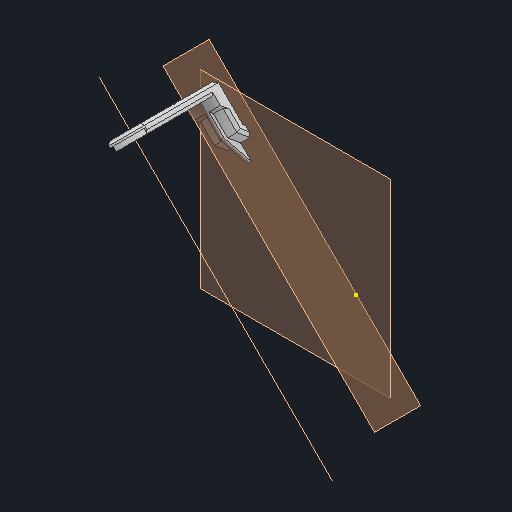
# Autodesk Inventor part: Venstre arm
Saved by Autodesk Inventor 2026.1 (Build 301233020, 233B)
## iProperties
Created: 2025-09-26
Part Number: Venstre arm
Material: Generic
Document SubType Name: Modeling
Designer: Malthe Sennels
Density: 1 g/cm^3
Appearance: Default
Author: Malthe Sennels
Autodesk Inventor part; units mm, degrees
ref_plane "YZ Plane" through (0, 0, 0) normal (1, 0, 0) x (0, 1, 0)
ref_plane "XZ Plane" through (0, 0, 0) normal (0, 1, 0) x (-1, 0, 0)
ref_plane "XY Plane" through (0, 0, 0) normal (0, 0, 1) x (1, 0, 0)
ref_plane "Work Plane1" through (0, 0, 0) normal (0, 0, 1) x (1, 0, 0)
sketch "Sketch1" plane through (0, 0, 0) normal (0, 0, 1) x (1, 0, 0)
  line L0 (-18.9164, 56.7911) -> (-19.9626, 56.4354) projected
  arc A0 (-12.4369, -46.9155) -> (-18.9164, 56.7911) centre (-94.7078, 0) ccw projected
  line L1 (-12.4369, -46.9155) -> (-25.0393, -34.3131) projected
  arc A1 (-25.0393, -34.3131) -> (-32.1104, -34.3131) centre (-28.5748, -37.8487) ccw projected
  line L2 (-32.1104, -34.3131) -> (-60.3946, -62.5974) projected
  arc A2 (-60.3946, -62.5974) -> (-60.3946, -69.6685) centre (-56.8591, -66.1329) ccw projected
  line L3 (-60.3946, -69.6685) -> (-47.7922, -82.2709) projected
  arc A3 (-141.6233, -82.2709) -> (-47.7922, -82.2709) centre (-94.7078, 0) ccw projected
  line L4 (-141.6233, -82.2709) -> (-129.0209, -69.6685) projected
  arc A4 (-129.0209, -69.6685) -> (-129.0209, -62.5974) centre (-132.5564, -66.1329) ccw projected
  line L5 (-129.0209, -62.5974) -> (-157.3052, -34.3131) projected
  arc A5 (-157.3052, -34.3131) -> (-164.3762, -34.3131) centre (-160.8407, -37.8487) ccw projected
  line L6 (-164.3762, -34.3131) -> (-176.9786, -46.9155) projected
  arc A6 (-176.9786, 46.9155) -> (-176.9786, -46.9155) centre (-94.7078, 0) ccw projected
  line L7 (-176.9786, 46.9155) -> (-164.3762, 34.3131) projected
  arc A7 (-164.3762, 34.3131) -> (-157.3052, 34.3131) centre (-160.8407, 37.8487) ccw projected
  line L8 (-157.3052, 34.3131) -> (-129.0209, 62.5974) projected
  arc A8 (-129.0209, 62.5974) -> (-129.0209, 69.6685) centre (-132.5564, 66.1329) ccw projected
  line L9 (-129.0209, 69.6685) -> (-141.6233, 82.2709) projected
  arc A9 (-37.9167, 75.7914) -> (-141.6233, 82.2709) centre (-94.7078, 0) ccw projected
  line L10 (-38.2723, 74.7452) -> (-37.9167, 75.7914) projected
  circle A10 centre (-138.2133, -64.7187) radius 2.25 projected
  circle A11 centre (-159.4265, -43.5055) radius 2.25 projected
  circle A12 centre (-159.4265, 43.5055) radius 2.25 projected
  circle A13 centre (-138.2133, 64.7187) radius 2.25 projected
  circle A14 centre (-51.2022, -64.7187) radius 2.25 projected
  circle A15 centre (-29.989, -43.5055) radius 2.25 projected
  line L11 (-141.6233, 82.2709) -> (-144.5624, 85.21)
  line L12 (-176.9786, 46.9155) -> (-179.9178, 49.8547)
  circle A16 centre (-94.7078, 0) radius 98.723 projected
  arc A17 (-19.9626, 56.4354) -> (-38.2723, 74.7452) centre (-94.7078, 0) ccw projected
  point P0 (0, 0)
  point P1 (-14.9261, 58.1475)
  point P2 (-36.5603, 79.7816)
  point P3 (-193.4308, 0)
  point P4 (-94.7078, -98.723)
  constraints: 4 end point, 2 point on circle, 1 parallel
extrude "Extrusion1" [suppressed]
chamfer "Chamfer1" [suppressed]
ref_plane "Work Plane2" through (-146.6986, 51.9908, -4) normal (0.7071068, 0.7071068, 0) x (0, 0, 1)
sketch "Sketch2" plane through (-146.6986, 51.9908, -4) normal (0.7071068, 0.7071068, 0) x (0, 0, 1)
  line L0 (8, 0) -> (8, -18.8747) projected
  line L1 (8, -18.8747) -> (8, -22.1969) projected
  line L2 (4, 5) -> (8, 5) projected
  line L3 (8, 5) -> (8, 0)
  line L4 (8, 5) -> (19.8525, -22.7909)
  line L5 (19.8525, -22.7909) -> (19.8525, -46.753)
  line L6 (19.8525, -46.753) -> (29.6486, -56.5491)
  line L7 (29.6486, -56.5491) -> (29.6486, -70.8342)
  line L8 (8, -22.1969) -> (9.8525, -24.0494)
  line L9 (8, -22.1969) -> (10.6198, -22.1969) construction
  line L10 (9.8525, -24.0494) -> (9.8525, -51.0381)
  line L11 (9.8525, -51.0381) -> (29.6486, -70.8342)
  line L12 (25.3635, -66.5491) -> (29.6486, -66.5491)
  line L13 (29.6486, -70.8342) -> (9.8525, -70.8342)
  line L14 (9.8525, -70.8342) -> (9.8525, -51.0381)
  line L15 (29.6486, -56.5491) -> (19.8525, -56.5491)
  line L16 (19.8525, -56.5491) -> (19.8525, -46.753)
  line L17 (29.6486, -66.5491) -> (9.8525, -66.5491)
  point P0 (4, 140.4946)
  point P1 (25.3635, -66.5491)
  dimension "d6" = 45
  dimension "d14" = 10
  dimension "d15" = 10
  constraints: 30 end point, 4 perpendicular, 3 point on line, 3 vertical, 2 collinear, 1 equal length, 1 horizontal, 1 parallel
  measures "d6" angle of L8 L9
  measures "d14" distance from line of L6.end L12
  measures "d15" distance between parallel lines of L5 L10
extrude "Extrusion2" add sketch "Sketch2" along normal mid plane 6 contours L3 L4 L5 L16 L15 L7 L12 L11 L10 L8 L1 L0 | L11 L17 L14
sketch "Sketch3" plane through (-144.5772, 54.1121, -4) normal (0.7071068, 0.7071068, 0) x (-0.7071068, 0.7071068, 0)
  line L0 (22.1969, 8) -> (24.0494, 9.8525) projected
  line L1 (24.0494, 9.8525) -> (66.5491, 9.8525) projected
  line L2 (51.0381, 9.8525) -> (66.5491, 25.3635) projected
  line L3 (56.5491, 29.6486) -> (46.753, 19.8525) projected
  line L4 (46.753, 19.8525) -> (43.753, 16.8525)
  line L5 (43.753, 16.8525) -> (21.1499, 16.8525)
  line L6 (21.1499, 16.8525) -> (12.2974, 8)
  line L7 (22.1499, 8) -> (-5, 8) projected
  line L8 (66.5491, 29.6486) -> (56.5491, 29.6486) projected
  line L9 (22.1499, 8) -> (12.2974, 8)
  line L10 (-5, 8) -> (22.1969, 8) projected
  line L11 (66.5491, 9.8525) -> (66.5491, 29.6486) projected
  line L12 (66.5491, 9.8525) -> (24.0494, 9.8525) projected
  line L13 (24.0494, 9.8525) -> (22.1969, 8) projected
  line L14 (22.1969, 8) -> (-5, 8) projected
  line L15 (-5, 8) -> (22.7909, 19.8525) projected
  line L16 (22.7909, 19.8525) -> (56.5491, 19.8525) projected
  line L17 (56.5491, 19.8525) -> (56.5491, 29.6486) projected
  line L18 (56.5491, 29.6486) -> (66.5491, 29.6486) projected
  line L19 (66.5491, 29.6486) -> (66.5491, 9.8525) projected
  point P0 (-140.4946, 4)
  point P1 (70.6913, 29.6486)
  point P2 (66.5491, 25.3635)
  point P3 (56.5491, 29.6486)
  dimension "d10" = 7
  dimension "d11" = 7
  constraints: 8 end point, 2 parallel, 1 collinear, 1 horizontal, 1 point on line, 1 other
  measures "d10" distance between parallel lines of L1 L5
  measures "d11" distance between parallel lines of L6 L0
extrude "Extrusion3" add sketch "Sketch3" along normal blind 18.2 contours L10 L7 L6 L5 L4 L16 L17 L8 L11 L2 L1 L0 | L2 L11 L1
mirror "Mirror1" about plane through (-146.6986, 51.9908, -4) normal (0.7071068, 0.7071068, 0) of "Extrusion3"
sketch "Sketch4" plane through (-171.6942, 106.9677, 25.6486) normal (0, 0, 1) x (0.7071068, 0.7071068, 0)
  point P0 (45.7685, -197.0437)
sketch "Sketch5" plane through (-181.028, 111.7761, 21.3635) normal (-0.7071068, 0.7071068, 0) x (-0.7071068, -0.7071068, 0)
  line L0 (-3.2, -15.511) -> (-3.2, 4.2851) projected
  line L1 (39.2, -15.511) -> (39.2, 4.2851) projected
  line L2 (39.2, 4.2851) -> (-3.2, 4.2851) projected
  line L3 (18, 4.2851) -> (18, 69.2851) construction
  circle A0 centre (18, 69.2851) radius 11
  arc A1 (39.2, 69.2851) -> (-3.2, 69.2851) centre (18, 69.2851) ccw
  line L4 (-3.2, 4.2851) -> (-3.2, 69.2851)
  line L5 (39.2, 4.2851) -> (39.2, 69.2851)
  line L6 (18, 51.2851) -> (4.8, 51.2851)
  line L7 (4.8, 51.2851) -> (-3.2, 59.2851)
  line L8 (18, 51.2851) -> (31.2, 51.2851)
  line L9 (31.2, 51.2851) -> (39.2, 59.2851)
  point P0 (-48.9685, -21.3635)
  point P1 (0, 0)
  point P2 (36, 0)
  dimension "d17" = 22
  dimension "d18" = 65
  dimension "d21" = 135
  dimension "d22" = 18
  dimension "d23" = 8
  constraints: 14 end point, 2 centre point, 2 coincident, 2 midpoint, 2 point on circle, 2 point on line, 2 symmetric about line, 2 vertical, 1 horizontal, 1 parallel, 1 tangent, 2 other
  measures "d17" diameter of A0
  measures "d18" distance of point (18, 4.285) L3.end
  measures "d21" angle of L6 L7
  measures "d22" distance from line of L3.end L6
  measures "d23" distance from line of L4 L6.end
extrude "Extrusion4" add sketch "Sketch5" against normal blind 10
chamfer "Chamfer2" distance 3 angle 45 6 edges at (-186.6848, 91.9771, 111.8486) (-171.6942, 106.9677, 53.2505) (-184.6359, 59.9468, 12.8525) (-154.6545, 89.9281, 12.8525) (-173.5146, 48.8256, 8.4262) (-143.5333, 78.8069, 8.4262)
sketch "Sketch7" plane through (-173.9569, 104.705, 21.3635) normal (0.7071068, -0.7071068, 0) x (0, 0, -1)
  circle A0 centre (-69.2851, -18) radius 11 projected
  line L0 (-69.2851, -18) -> (-10.1777, -18) construction
  line L1 (-51.2851, -18) -> (-51.2851, -30)
  line L2 (-51.2851, -30) -> (-57.2851, -36)
  line L3 (-69.2851, -36) -> (-3.0425, -36) projected
  line L4 (-51.2851, -18) -> (-51.2851, -6)
  line L5 (-51.2851, -6) -> (-57.2851, 0)
  line L6 (-69.2851, -39.2) -> (-69.2851, -36.2) projected
  arc A1 (-69.2851, 0.2) -> (-69.2851, -36.2) centre (-69.2851, -18) ccw projected
  line L7 (-69.2851, 3.2) -> (-69.2851, 0.2) projected
  arc A2 (-69.2851, 3.2) -> (-69.2851, -39.2) centre (-69.2851, -18) ccw projected
  line L8 (5.511, 3.2) -> (-69.2851, 3.2) projected
  point P0 (21.3635, 48.9685)
  point P1 (-3.0425, 0)
  point P2 (-69.2851, -36)
  dimension "d32" = 135
  dimension "d33" = 6
  dimension "d34" = 18
  constraints: 10 end point, 2 point on line, 2 symmetric about line, 1 horizontal, 1 vertical, 1 other
  measures "d32" angle of L1 L2
  measures "d33" distance from line of L3 L1.end
  measures "d34" distance of L0.start L1.start
extrude "Extrusion6" cut sketch "Sketch7" against normal blind 5 contours A2 L7 A1 L6
ref_plane "Work Plane3" through (-146.6986, 51.9908, -4) normal (0.7071068, 0.7071068, 0) x (0, 0, 1)
sketch "Sketch8" plane through (-146.6986, 51.9908, -4) normal (0.7071068, 0.7071068, 0) x (0, 0, 1)
  line L0 (105.6486, -66.5491) -> (83.6486, -66.5491) projected
  line L1 (105.6486, -61.5491) -> (83.6486, -61.5491) projected
  circle A0 centre (105.4486, -61.5491) radius 2.325
  circle A1 centre (105.4486, -61.5491) radius 2.25 construction
  line L2 (94.6486, -140.0947) -> (94.6486, 226.3244) projected
  point P0 (4, 140.4946)
  dimension "d37" = 4.65
  dimension "d38" = 4.5
  dimension "d39" = 0.2
  constraints: 2 centre point, 1 coincident, 1 point on line
  measures "d37" diameter of A0
  measures "d38" diameter of A1
  measures "d39" distance of L1.start A0.centre
revolve "Revolution1" cut sketch "Sketch8" angle 360 about axis through (-193.7559, 99.0481, 90.6486) along (0.7071068, -0.7071068, 0)
chamfer "Chamfer3" distance 1.5 angle 45 1 edges at (-185.9777, 106.8263, 90.6486)
sketch "Sketch9" plane through (-177.4924, 108.2405, 21.3635) normal (0.7071068, -0.7071068, 0) x (-0.7071068, -0.7071068, 0)
  line L0 (30, -51.2851) -> (36, -57.2851) projected
  line L1 (33, -54.2851) -> (33, -61.3562) construction
  line L2 (33, -54.2851) -> (40.0711, -54.2851) construction
  circle A0 centre (33, -61.3562) radius 1.75
  line L3 (6, -51.2851) -> (30, -51.2851) projected
  line L4 (18, -51.2851) -> (18, -96.7348) construction
  circle A1 centre (3, -61.3562) radius 1.75
  point P0 (-48.9685, 21.3635)
  dimension "d44" = 90
  dimension "d45" = 3.5
  dimension "d46" = 5
  constraints: 6 end point, 2 centre point, 2 coincident, 2 midpoint, 2 symmetric about line, 1 horizontal, 1 perpendicular, 1 vertical, 1 other
  measures "d44" angle of L1 L2
  measures "d45" diameter of A0
  measures "d46" distance from line of L0 L1.end
extrude "Extrusion7" cut sketch "Sketch9" against normal through all
sketch "Sketch10" plane through (-206.4838, 86.3202, 21.3635) normal (-0.7071068, 0.7071068, 0) x (-0.7071068, -0.7071068, 0)
  line L0 (-30.75, 59.1062) -> (-35.25, 59.1062)
  line L1 (-35.25, 59.1062) -> (-35.25, 63.6062)
  line L2 (-35.25, 63.6062) -> (-30.75, 63.6062)
  line L3 (-30.75, 63.6062) -> (-30.75, 59.1062)
  circle A0 centre (-33, 61.3562) radius 1.75 construction
  line L4 (-30.75, 59.1062) -> (-35.25, 63.6062) construction
  line L5 (-35.25, 59.1062) -> (-30.75, 63.6062) construction
  line L6 (-0.75, 59.1062) -> (-5.25, 59.1062)
  line L7 (-5.25, 59.1062) -> (-5.25, 63.6062)
  line L8 (-5.25, 63.6062) -> (-0.75, 63.6062)
  line L9 (-0.75, 63.6062) -> (-0.75, 59.1062)
  circle A1 centre (-3, 61.3562) radius 1.75 construction
  line L10 (-0.75, 59.1062) -> (-5.25, 63.6062) construction
  line L11 (-5.25, 59.1062) -> (-0.75, 63.6062) construction
  point P0 (-84.9685, -21.3635)
  dimension "d49" = 4.5
  dimension "d50" = 4.5
  dimension "d51" = 4.5
  dimension "d52" = 4.5
  constraints: 24 end point, 4 midpoint, 4 parallel, 2 horizontal, 2 perpendicular
  measures "d49" distance of L1.end L2.end
  measures "d50" distance of L0.end L1.end
  measures "d51" distance of L7.end L8.end
  measures "d52" distance of L6.end L7.end
extrude "Extrusion8" cut sketch "Sketch10" against normal blind 3
chamfer "Chamfer4" distance 3 angle 45 3 edges at (-208.7466, 84.0575, 48.2505) (-193.7559, 99.0481, 111.8486) (-178.7652, 114.0388, 48.2505)
ref_plane "Work Plane4" through (-146.6986, 51.9908, -4) normal (0.7071068, 0.7071068, 0) x (0, 0, 1)
sketch "Sketch11" plane through (-146.6986, 51.9908, -4) normal (0.7071068, 0.7071068, 0) x (0, 0, 1)
  line L0 (5, -25.1969) -> (8, -22.1969) projected
  line L1 (5, -25.1969) -> (9.8525, -51.0381) construction
  line L2 (9.8525, -24.0494) -> (9.8525, -63.5491) projected
  line L3 (8, -22.1969) -> (9.8525, -24.0494) projected
  line L4 (4.0696, -25.6606) -> (10.8525, -61.7819)
  line L5 (10.8525, -61.7819) -> (10.8525, -23.6352)
  line L6 (10.8525, -23.6352) -> (8, -20.7827)
  line L7 (8, -20.7827) -> (4.2929, -24.4898)
  line L8 (9.8525, -51.0381) -> (22.3635, -63.5491) projected
  line L9 (5, -25.1969) -> (4.7764, -24.0063) construction
  arc A0 (9.8525, -51.0381) -> (4.5973, -24.1854) centre (-61.3805, -51.0381) ccw
  line L10 (5, -25.1969) -> (5, -21.9791) projected
  line L11 (5, -25.1969) -> (5, -63.5491)
  line L12 (5, -63.5491) -> (9.8525, -63.5491)
  point P0 (4, 140.4946)
  point P1 (8, -19.8198)
  point P2 (5, -25.1969)
  point P3 (10.8525, -52.0381)
  dimension "d58" = 1
  constraints: 16 end point, 4 point on circle, 3 point on line, 2 collinear, 1 centre point, 1 perpendicular, 1 tangent, 3 other
  measures "d58" distance between parallel lines of L2 L5
extrude "Extrusion9" add sketch "Sketch11" along normal mid plane 6 contours L0 L3 L2 A0 | A0 L2 L4 L11 | L4 L2 L12 L11
chamfer "Chamfer5" [suppressed]
chamfer "Chamfer6" distance 3 angle 45 1 edges at (-193.7559, 99.0481, 5.8525)
chamfer "Chamfer7" distance 4 angle 45 1 edges at (-191.6346, 96.9268, 1)
sketch "Sketch13" plane through (-199.5542, 79.1077, 90.6486) normal (0.7071068, -0.7071068, 0) x (-0.7071068, -0.7071068, 0)
  line L0 (0, 74.7961) -> (-36.4, 74.7961) projected
  line L1 (-36.4, 74.7961) -> (-18.2, 74.7961)
  line L2 (-18.2, 74.7961) -> (-18.2, 53.6461)
  circle A0 centre (-18.2, 53.6461) radius 2.5
  point P0 (-85.1685, 90.6486)
  dimension "d72" = 18.2
  dimension "d73" = 21.15
  dimension "d74" = 5
  constraints: 4 end point, 1 centre point, 1 coincident, 1 midpoint, 1 perpendicular
  measures "d72" distance of L0.end L1.end
  measures "d73" distance of L1.end L2.end
  measures "d74" diameter of A0
extrude "Extrusion11" cut sketch "Sketch13" against normal blind 13
sketch "Sketch14" plane through (-206.6252, 86.1788, 8.8525) normal (-0.7071068, 0.7071068, 0) x (-0.7071068, -0.7071068, 0)
  circle A0 centre (-2.7, 43.65) radius 1.5
  circle A1 centre (-2.7, 12.65) radius 1.5
  circle A2 centre (-33.7, 12.65) radius 1.5
  circle A3 centre (-33.7, 43.65) radius 1.5
  point P0 (-85.1685, -8.8525)
  constraints: 4 centre point, 8 other
extrude "Extrusion12" cut sketch "Sketch14" against normal blind 13
sketch "Sketch15" plane through (-206.6252, 86.1788, 8.8525) normal (-0.7071068, 0.7071068, 0) x (-0.7071068, -0.7071068, 0)
  circle A0 centre (-33.7, 43.65) radius 1.5 projected
  circle A1 centre (-2.7, 43.65) radius 1.5 projected
  circle A2 centre (-2.7, 12.65) radius 1.5 projected
  circle A3 centre (-33.7, 12.65) radius 1.5 projected
  circle A4 centre (-33.7, 43.65) radius 3
  circle A5 centre (-2.7, 43.65) radius 3
  circle A6 centre (-33.7, 12.65) radius 3
  circle A7 centre (-2.7, 12.65) radius 3
  point P0 (-85.1685, -8.8525)
  dimension "d79" = 6
  dimension "d80" = 6
  dimension "d81" = 6
  dimension "d82" = 6
  constraints: 4 centre point, 4 coincident
  measures "d79" diameter of A4
  measures "d80" diameter of A5
  measures "d81" diameter of A6
  measures "d82" diameter of A7
extrude "Extrusion13" cut sketch "Sketch15" against normal blind 3 contours A0 | A1 | A2 | A3 | A4 | A5 | A6 | A7
body "Solid1"
